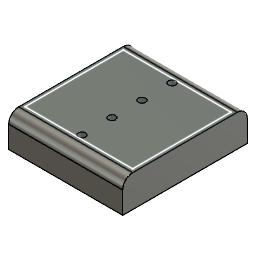
Battery pack (Autodesk Fusion 360 design; units mm, degrees)
Autodesk Fusion 360 part; units mm, degrees
sketch "Sketch1" plane through (0, 0, 0) normal (0, 1, 0) x (1, 0, 0)
  line L0 (0, 0) -> (57, 0)
  line L1 (57, 0) -> (57, 62.3)
  line L2 (57, 62.3) -> (0, 62.3)
  line L3 (0, 62.3) -> (0, 0)
  dimension "d1" = 57
  dimension "d2" = 62.3
  constraint horizontal L0
  constraint vertical L1
  constraint horizontal L2
  constraint vertical L3
  constraint coincident L0.start L3.end
  measures "d1" distance of L0.start L0.end
  measures "d2" distance of L0.start L2.end
extrude "Extrude1" add sketch "Sketch1" along normal blind 16
fillet "Fillet1" radius 5 2 edges at (28.5, 16, 0) (28.5, 16, -62.3)
sketch "Sketch2" plane through (0, 16, 0) normal (0, 1, 0) x (-1, 0, 0)
  line L0 (-57, -57.3) -> (0, -57.3)
  line L1 (0, -57.3) -> (0, -5)
  line L2 (0, -5) -> (-57, -5)
  line L3 (-57, -5) -> (-57, -57.3)
  line L4 (-55.4, -6.6) -> (-1.6, -6.6)
  line L5 (-1.6, -6.6) -> (-1.6, -55.7)
  line L6 (-1.6, -55.7) -> (-55.4, -55.7)
  line L7 (-55.4, -55.7) -> (-55.4, -6.6)
  dimension "d7" = 1.6
  dimension "d8" = 1.6
  dimension "d9" = 1.6
  dimension "d10" = 1.6
  constraint horizontal L4
  constraint vertical L5
  constraint horizontal L6
  constraint vertical L7
  measures "d7" distance of L1 L5
  measures "d8" distance of L3 L7
  measures "d9" distance of L0 L6
  measures "d10" distance of L2 L4
sketch "Sketch3" plane through (0, 0, 0) normal (0, -1, 0) x (1, 0, 0)
  line L0 (0, 0) -> (0, -62.3)
  line L1 (0, -62.3) -> (57, -62.3)
  line L2 (57, -62.3) -> (57, 0)
  line L3 (57, 0) -> (0, 0)
  circle A0 centre (28, -53.7) radius 1.8
  circle A1 centre (28, -38.67) radius 1.8
  circle A2 centre (28, -23.64) radius 1.8
  circle A3 centre (28, -8.61) radius 1.8
  dimension "d11" = 3.6
  dimension "d12" = 28
  dimension "d13" = 8.6
  dimension "d16" = 0
  dimension "d17" = 15.03
  dimension "d18" = 8.61
  measures "d11" diameter of A0
  measures "d12" distance of L0 A0.centre
  measures "d13" distance of L1 A0.centre
  measures "d18" distance of L3 A3.centre
extrude "Extrude2" cut sketch "Sketch3" against normal blind 45 contours A0 | A1 | A2 | A3
equation "d9 = d7"
equation "d10 = d9"
equation "d13 = 6.8 mm + ( ( 3.6 / 2 ) * 1 mm )"
equation "d17 = 11.43 mm + 3.6 mm"
